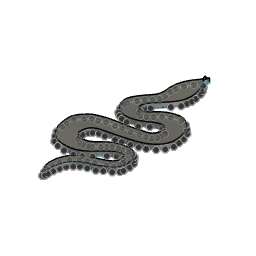
Snakegame Enclosure v3.1 v1 (Autodesk Fusion 360 archive; units mm, degrees)
design "Snake Logo"
Autodesk Fusion 360 part; units mm, degrees
note: some values were not read from the file. Chosen so that the rebuilt part matches the saved one: that a step has no effect; which face or edge a step refers to.
mesh "Mesh1" [no effect]
sketch "Sketch4" plane through (0, 0, 0) normal (0, 0, 1) x (1, 0, 0)
  line L0 (-0.7146, -1.2616) -> (-1.3572, -2.1185)
  line L1 (-1.3572, -2.1185) -> (-2.1784, -3.5109)
  line L2 (-2.1784, -3.5109) -> (-2.6069, -4.939)
  line L3 (-2.6069, -4.939) -> (-2.6426, -6.0815)
  line L4 (-2.6426, -6.0815) -> (-2.3569, -7.5811)
  line L5 (-2.3569, -7.5811) -> (-2.464, -8.6522)
  line L6 (-2.464, -8.6522) -> (-3.071, -9.6519)
  line L7 (-3.071, -9.6519) -> (-3.8922, -10.5445)
  line L8 (-3.8922, -10.5445) -> (-4.6063, -11.5442)
  line L9 (-4.6063, -11.5442) -> (-5.331, -12.983)
  line L10 (-5.331, -12.983) -> (-5.3916, -13.7466)
  line L11 (-5.3916, -13.7466) -> (-4.997, -14.9317)
  line L12 (-4.997, -14.9317) -> (-4.4158, -15.8778)
  line L13 (-4.4158, -15.8778) -> (-3.6886, -16.3618)
  line L14 (-3.6886, -16.3618) -> (-2.866, -16.6978)
  line L15 (-2.866, -16.6978) -> (-1.6605, -16.8088)
  line L16 (-1.6605, -16.8088) -> (0.4422, -16.3213)
  line L17 (0.4422, -16.3213) -> (1.8168, -15.1431)
  line L18 (1.8168, -15.1431) -> (3.5056, -14.0434)
  line L19 (3.5056, -14.0434) -> (4.4481, -14.4361)
  line L20 (4.4481, -14.4361) -> (4.8801, -14.7896)
  line L21 (4.8801, -14.7896) -> (4.9587, -15.6929)
  line L22 (4.9587, -15.6929) -> (4.8409, -16.4784)
  line L23 (4.8409, -16.4784) -> (4.3303, -17.2246)
  line L24 (4.3303, -17.2246) -> (3.427, -17.6173)
  line L25 (3.427, -17.6173) -> (2.131, -17.7744)
  line L26 (2.131, -17.7744) -> (0.7462, -18.3531)
  line L27 (0.7462, -18.3531) -> (-0.9311, -18.4963)
  line L28 (-0.9311, -18.4963) -> (-2.2118, -18.8395)
  line L29 (-2.2118, -18.8395) -> (-3.9449, -19.1238)
  line L30 (-3.9449, -19.1238) -> (-5.0863, -19.7538)
  line L31 (-5.0863, -19.7538) -> (-6.2013, -20.0165)
  line L32 (-6.2013, -20.0165) -> (-6.9345, -21.0054)
  line L33 (-6.9345, -21.0054) -> (-8.073, -22.2076)
  line L34 (-8.073, -22.2076) -> (-8.1115, -23.7858)
  line L35 (-8.1115, -23.7858) -> (-7.919, -24.902)
  line L36 (-7.919, -24.902) -> (-7.6303, -26.4725)
  line L37 (-7.6303, -26.4725) -> (-6.9105, -27.5311)
  line L38 (-6.9105, -27.5311) -> (-5.979, -28.5896)
  line L39 (-5.979, -28.5896) -> (-4.7511, -29.0554)
  line L40 (-4.7511, -29.0554) -> (-3.1845, -29.2671)
  line L41 (-3.1845, -29.2671) -> (-1.3638, -29.013)
  line L42 (-1.3638, -29.013) -> (-0.0512, -28.3355)
  line L43 (-0.0512, -28.3355) -> (1.1767, -27.277)
  line L44 (1.1767, -27.277) -> (2.6163, -25.541)
  line L45 (2.6163, -25.541) -> (3.8018, -24.5248)
  line L46 (3.8018, -24.5248) -> (5.0297, -24.2708)
  line L47 (5.0297, -24.2708) -> (5.5802, -24.5672)
  line L48 (5.5802, -24.5672) -> (5.8342, -25.1176)
  line L49 (5.8342, -25.1176) -> (5.8342, -25.9221)
  line L50 (5.8342, -25.9221) -> (5.4955, -26.8536)
  line L51 (5.4955, -26.8536) -> (4.437, -27.4464)
  line L52 (4.437, -27.4464) -> (2.701, -28.2932)
  line L53 (2.701, -28.2932) -> (1.4731, -28.7166)
  line L54 (1.4731, -28.7166) -> (0.4569, -29.4364)
  line L55 (0.4569, -29.4364) -> (-0.7146, -30.5373)
  line L56 (-0.7146, -30.5373) -> (-1.4062, -32.0616)
  line L57 (-1.4062, -32.0616) -> (-1.6179, -33.4589)
  line L58 (-1.6179, -33.4589) -> (-1.5755, -34.7291)
  line L59 (-1.5755, -34.7291) -> (-1.2368, -35.6606)
  line L60 (-1.2368, -35.6606) -> (-0.7146, -36.5842)
  line L61 (-0.7146, -36.5842) -> (-0.472, -36.2071)
  line L62 (-0.472, -36.2071) -> (-0.472, -35.5521)
  line L63 (-0.472, -35.5521) -> (-0.3926, -34.4802)
  line L64 (-0.3926, -34.4802) -> (-0.1941, -33.2893)
  line L65 (-0.1941, -33.2893) -> (0.1831, -32.1778)
  line L66 (0.1831, -32.1778) -> (0.9175, -31.3243)
  line L67 (0.9175, -31.3243) -> (1.6717, -30.5899)
  line L68 (1.6717, -30.5899) -> (2.8229, -30.0738)
  line L69 (2.8229, -30.0738) -> (4.2124, -29.5776)
  line L70 (4.2124, -29.5776) -> (5.1651, -28.863)
  line L71 (5.1651, -28.863) -> (6.3957, -28.0889)
  line L72 (6.3957, -28.0889) -> (7.1897, -27.1957)
  line L73 (7.1897, -27.1957) -> (7.3683, -26.5804)
  line L74 (7.3683, -26.5804) -> (7.4239, -25.2466)
  line L75 (7.4239, -25.2466) -> (7.1837, -24.0676)
  line L76 (7.1837, -24.0676) -> (6.5724, -23.3689)
  line L77 (6.5724, -23.3689) -> (5.9392, -22.6921)
  line L78 (5.9392, -22.6921) -> (5.1969, -22.4301)
  line L79 (5.1969, -22.4301) -> (4.3672, -22.4082)
  line L80 (4.3672, -22.4082) -> (3.1882, -22.6702)
  line L81 (3.1882, -22.6702) -> (2.4895, -22.8667)
  line L82 (2.4895, -22.8667) -> (1.5506, -23.2597)
  line L83 (1.5506, -23.2597) -> (0.8738, -23.8492)
  line L84 (0.8738, -23.8492) -> (0.2624, -24.5043)
  line L85 (0.2624, -24.5043) -> (-0.7146, -25.4082)
  line L86 (-0.7146, -25.4082) -> (-1.2135, -25.7684)
  line L87 (-1.2135, -25.7684) -> (-2.1262, -26.0086)
  line L88 (-2.1262, -26.0086) -> (-2.9908, -26.0326)
  line L89 (-2.9908, -26.0326) -> (-3.9034, -25.5042)
  line L90 (-3.9034, -25.5042) -> (-4.2156, -24.9518)
  line L91 (-4.2156, -24.9518) -> (-4.1196, -24.1593)
  line L92 (-4.1196, -24.1593) -> (-3.9034, -23.1746)
  line L93 (-3.9034, -23.1746) -> (-3.4231, -22.6702)
  line L94 (-3.4231, -22.6702) -> (-2.5585, -22.1178)
  line L95 (-2.5585, -22.1178) -> (-1.3816, -21.9737)
  line L96 (-1.3816, -21.9737) -> (0.4094, -21.4817)
  line L97 (0.4094, -21.4817) -> (1.5874, -21.1661)
  line L98 (1.5874, -21.1661) -> (3.1374, -20.7659)
  line L99 (3.1374, -20.7659) -> (4.5173, -20.3203)
  line L100 (4.5173, -20.3203) -> (5.6912, -19.7931)
  line L101 (5.6912, -19.7931) -> (6.9704, -18.8732)
  line L102 (6.9704, -18.8732) -> (7.8817, -17.7419)
  line L103 (7.8817, -17.7419) -> (8.3309, -16.3153)
  line L104 (8.3309, -16.3153) -> (8.204, -15.0393)
  line L105 (8.204, -15.0393) -> (8.0006, -13.7897)
  line L106 (8.0006, -13.7897) -> (7.3904, -12.3657)
  line L107 (7.3904, -12.3657) -> (6.5185, -11.552)
  line L108 (6.5185, -11.552) -> (5.4724, -10.7674)
  line L109 (5.4724, -10.7674) -> (4.2227, -10.5058)
  line L110 (4.2227, -10.5058) -> (2.3919, -11.058)
  line L111 (2.3919, -11.058) -> (1.2295, -11.8136)
  line L112 (1.2295, -11.8136) -> (0.3286, -12.8016)
  line L113 (0.3286, -12.8016) -> (-0.3979, -13.6153)
  line L114 (-0.3979, -13.6153) -> (-1.3569, -14.0803)
  line L115 (-1.3569, -14.0803) -> (-2.1415, -13.7025)
  line L116 (-2.1415, -13.7025) -> (-2.4321, -13.1213)
  line L117 (-2.4321, -13.1213) -> (-2.2578, -12.0461)
  line L118 (-2.2578, -12.0461) -> (-1.7056, -11.4358)
  line L119 (-1.7056, -11.4358) -> (0.3577, -8.9714)
  line L120 (0.3577, -8.9714) -> (1.3167, -7.6288)
  line L121 (1.3167, -7.6288) -> (1.4765, -6.542)
  line L122 (1.4765, -6.542) -> (1.6364, -5.583)
  line L123 (1.6364, -5.583) -> (1.5405, -4.624)
  line L124 (1.5405, -4.624) -> (1.2208, -3.2494)
  line L125 (1.2208, -3.2494) -> (0.8372, -2.3863)
  line L126 (0.8372, -2.3863) -> (0.2298, -1.5871)
  line L127 (0.2298, -1.5871) -> (-0.1538, -1.2616)
  spline S0 degree 5 poles (-0.7146, -1.2616) (-1.3572, -2.1185) (-2.1784, -3.5109) (-2.6069, -4.939) (-2.6426, -6.0815) (-2.3569, -7.5811) (-2.464, -8.6522) (-3.071, -9.6519) (-3.8922, -10.5445) (-4.6063, -11.5442) (-5.331, -12.983) (-5.3916, -13.7466) (-4.997, -14.9317) (-4.4158, -15.8778) (-3.6886, -16.3618) (-2.866, -16.6978) (-1.6605, -16.8088) (0.4422, -16.3213) (1.8168, -15.1431) (3.5056, -14.0434) (4.4481, -14.4361) (4.8801, -14.7896) (4.9587, -15.6929) (4.8409, -16.4784) (4.3303, -17.2246) (3.427, -17.6173) (2.131, -17.7744) (0.7462, -18.3531) (-0.9311, -18.4963) (-2.2118, -18.8395) (-3.9449, -19.1238) (-5.0863, -19.7538) (-6.2013, -20.0165) (-6.9345, -21.0054) (-8.073, -22.2076) (-8.1115, -23.7858) (-7.919, -24.902) (-7.6303, -26.4725) (-6.9105, -27.5311) (-5.979, -28.5896) (-4.7511, -29.0554) (-3.1845, -29.2671) (-1.3638, -29.013) (-0.0512, -28.3355) (1.1767, -27.277) (2.6163, -25.541) (3.8018, -24.5248) (5.0297, -24.2708) (5.5802, -24.5672) (5.8342, -25.1176) (5.8342, -25.9221) (5.4955, -26.8536) (4.437, -27.4464) (2.701, -28.2932) (1.4731, -28.7166) (0.4569, -29.4364) (-0.7146, -30.5373) (-1.4062, -32.0616) (-1.6179, -33.4589) (-1.5755, -34.7291) (-1.2368, -35.6606) (-0.7146, -36.5842) (-0.472, -36.2071) (-0.472, -35.5521) (-0.3926, -34.4802) (-0.1941, -33.2893) (0.1831, -32.1778) (0.9175, -31.3243) (1.6717, -30.5899) (2.8229, -30.0738) (4.2124, -29.5776) (5.1651, -28.863) (6.3957, -28.0889) (7.1897, -27.1957) (7.3683, -26.5804) (7.4239, -25.2466) (7.1837, -24.0676) (6.5724, -23.3689) (5.9392, -22.6921) (5.1969, -22.4301) (4.3672, -22.4082) (3.1882, -22.6702) (2.4895, -22.8667) (1.5506, -23.2597) (0.8738, -23.8492) (0.2624, -24.5043) (-0.7146, -25.4082) (-1.2135, -25.7684) (-2.1262, -26.0086) (-2.9908, -26.0326) (-3.9034, -25.5042) (-4.2156, -24.9518) (-4.1196, -24.1593) (-3.9034, -23.1746) (-3.4231, -22.6702) (-2.5585, -22.1178) (-1.3816, -21.9737) (0.4094, -21.4817) (1.5874, -21.1661) (3.1374, -20.7659) (4.5173, -20.3203) (5.6912, -19.7931) (6.9704, -18.8732) (7.8817, -17.7419) (8.3309, -16.3153) (8.204, -15.0393) (8.0006, -13.7897) (7.3904, -12.3657) (6.5185, -11.552) (5.4724, -10.7674) (4.2227, -10.5058) (2.3919, -11.058) (1.2295, -11.8136) (0.3286, -12.8016) (-0.3979, -13.6153) (-1.3569, -14.0803) (-2.1415, -13.7025) (-2.4321, -13.1213) (-2.2578, -12.0461) (-1.7056, -11.4358) (0.3577, -8.9714) (1.3167, -7.6288) (1.4765, -6.542) (1.6364, -5.583) (1.5405, -4.624) (1.2208, -3.2494) (0.8372, -2.3863) (0.2298, -1.5871) (-0.1538, -1.2616) knots 0 0 0 0 0 0 0.00806452 0.01612903 0.02419355 0.03225806 0.04032258 0.0483871 0.05645161 0.06451613 0.07258065 0.08064516 0.08870968 0.09677419 0.10483871 0.11290323 0.12096774 0.12903226 0.13709677 0.14516129 0.15322581 0.16129032 0.16935484 0.17741935 0.18548387 0.19354839 0.2016129 0.20967742 0.21774194 0.22580645 0.23387097 0.24193548 0.25 0.25806452 0.26612903 0.27419355 0.28225806 0.29032258 0.2983871 0.30645161 0.31451613 0.32258065 0.33064516 0.33870968 0.34677419 0.35483871 0.36290323 0.37096774 0.37903226 0.38709677 0.39516129 0.40322581 0.41129032 0.41935484 0.42741935 0.43548387 0.44354839 0.4516129 0.45967742 0.46774194 0.47580645 0.48387097 0.49193548 0.5 0.50806452 0.51612903 0.52419355 0.53225806 0.54032258 0.5483871 0.55645161 0.56451613 0.57258065 0.58064516 0.58870968 0.59677419 0.60483871 0.61290323 0.62096774 0.62903226 0.63709677 0.64516129 0.65322581 0.66129032 0.66935484 0.67741935 0.68548387 0.69354839 0.7016129 0.70967742 0.71774194 0.72580645 0.73387097 0.74193548 0.75 0.75806452 0.76612903 0.77419355 0.78225806 0.79032258 0.7983871 0.80645161 0.81451613 0.82258065 0.83064516 0.83870968 0.84677419 0.85483871 0.86290323 0.87096774 0.87903226 0.88709677 0.89516129 0.90322581 0.91129032 0.91935484 0.92741935 0.93548387 0.94354839 0.9516129 0.95967742 0.96774194 0.97580645 0.98387097 0.99193548 1 1 1 1 1 1
  line L128 (-0.1538, -1.2616) -> (-0.2247, -1.0744)
  line L129 (-0.2247, -1.0744) -> (0, 0)
  line L130 (0, 0) -> (-0.3558, -0.4855)
  line L131 (-0.3558, -0.4855) -> (-0.8014, 0)
  line L132 (-0.8014, 0) -> (-0.7582, -0.3591)
  line L133 (-0.7582, -0.3591) -> (-0.5786, -0.8214)
  line L134 (-0.5786, -0.8214) -> (-0.5945, -1.0641)
  line L135 (-0.5945, -1.0641) -> (-0.7146, -1.2616)
extrude "Extrude1" add sketch "Sketch4" along normal blind 1 contours L4 L5 L6 L7 L17 L18 L19 L20 L21 L22 L23 L24 L25 L26 L27 L28 L29 L30 L31 L32 L33 L44 L45 L46 L47 L48 L49 L50 L51 L52 L53 L62 L63 L64 L65 L66 L67 L68 L69 L70 L71 L84 L85 L86 L87 L88 L89 L90 L91 L92 L93 L94 L95 L97 L98 L113 L114 L115 L116 L117 L118 L119 S0 L128 L129 L130 L131 L132 L133 L134 L135 | L4 L5 L6 L7 S0 | L17 L18 L19 L20 L21 L22 L23 L24 L25 S0 | L26 L27 S0 | L28 L29 S0 | L30 L31 S0 | L113 L114 L115 L116 L117 L118 L119 S0 | L32 L33 S0 | L97 L98 S0 | L44 L45 L46 L47 L48 L49 L50 L51 L52 L53 S0 | L84 L85 L86 L87 L88 L89 L90 L91 L92 L93 L94 L95 S0 | L62 L63 L64 L65 L66 L67 L68 L69 S0 | L70 L71 S0
